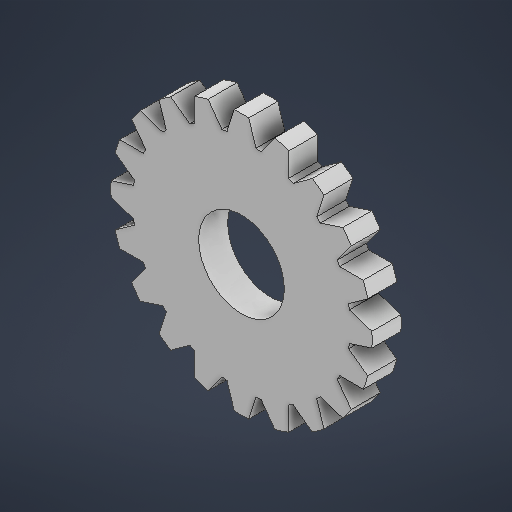
# Autodesk Inventor part: Engrenagem
Saved by Autodesk Inventor 2026.2 (Build 302298010, 298A)
## iProperties
Created: 2026-04-22
Part Number: Engrenagem
Material: Generic
Document SubType Name: Modeling
Designer: mrcm
Density: 1 g/cm^3
Appearance: Default
Author: mrcm
Autodesk Inventor part; units mm, degrees
ref_plane "YZ Plane" through (0, 0, 0) normal (1, 0, 0) x (0, 1, 0)
ref_plane "XZ Plane" through (0, 0, 0) normal (0, 1, 0) x (-1, 0, 0)
ref_plane "XY Plane" through (0, 0, 0) normal (0, 0, 1) x (1, 0, 0)
sketch "Sketch1" plane through (0, 0, 0) normal (0, 0, 1) x (1, 0, 0)
  arc A0 (12.7, 228.2469) -> (-12.7, 228.2469) centre (0, 0) ccw
  line L0 (-25.4, 188.7991) -> (-12.7, 228.2469)
  line L1 (12.7, 228.2469) -> (25.4, 188.7991)
  arc A1 (-58.4538, 221.0003) -> (-82.6106, 213.1512) centre (0, 0) ccw
  line L2 (-82.499, 171.7096) -> (-82.6106, 213.1512)
  line L3 (-58.4538, 221.0003) -> (-34.1853, 187.4076)
  arc A2 (-123.8857, 192.1205) -> (-144.4347, 177.1908) centre (0, 0) ccw
  line L4 (-131.5223, 137.8119) -> (-144.4347, 177.1908)
  line L5 (-123.8857, 192.1205) -> (-90.4243, 167.6714)
  arc A3 (-177.1908, 144.4347) -> (-192.1205, 123.8857) centre (0, 0) ccw
  line L6 (-167.6714, 90.4243) -> (-192.1205, 123.8857)
  line L7 (-177.1908, 144.4347) -> (-137.8119, 131.5223)
  arc A4 (-213.1512, 82.6106) -> (-221.0003, 58.4538) centre (0, 0) ccw
  line L8 (-187.4076, 34.1853) -> (-221.0003, 58.4538)
  line L9 (-213.1512, 82.6106) -> (-171.7096, 82.499)
  arc A5 (-228.2469, 12.7) -> (-228.2469, -12.7) centre (0, 0) ccw
  line L10 (-188.7991, -25.4) -> (-228.2469, -12.7)
  line L11 (-228.2469, 12.7) -> (-188.7991, 25.4)
  arc A6 (-221.0003, -58.4538) -> (-213.1512, -82.6106) centre (0, 0) ccw
  line L12 (-171.7096, -82.499) -> (-213.1512, -82.6106)
  line L13 (-221.0003, -58.4538) -> (-187.4076, -34.1853)
  arc A7 (-192.1205, -123.8857) -> (-177.1908, -144.4347) centre (0, 0) ccw
  line L14 (-137.8119, -131.5223) -> (-177.1908, -144.4347)
  line L15 (-192.1205, -123.8857) -> (-167.6714, -90.4243)
  arc A8 (-144.4347, -177.1908) -> (-123.8857, -192.1205) centre (0, 0) ccw
  line L16 (-90.4243, -167.6714) -> (-123.8857, -192.1205)
  line L17 (-144.4347, -177.1908) -> (-131.5223, -137.8119)
  arc A9 (-82.6106, -213.1512) -> (-58.4538, -221.0003) centre (0, 0) ccw
  line L18 (-34.1853, -187.4076) -> (-58.4538, -221.0003)
  line L19 (-82.6106, -213.1512) -> (-82.499, -171.7096)
  arc A10 (-12.7, -228.2469) -> (12.7, -228.2469) centre (0, 0) ccw
  line L20 (25.4, -188.7991) -> (12.7, -228.2469)
  line L21 (-12.7, -228.2469) -> (-25.4, -188.7991)
  arc A11 (58.4538, -221.0003) -> (82.6106, -213.1512) centre (0, 0) ccw
  line L22 (82.499, -171.7096) -> (82.6106, -213.1512)
  line L23 (58.4538, -221.0003) -> (34.1853, -187.4076)
  arc A12 (123.8857, -192.1205) -> (144.4347, -177.1908) centre (0, 0) ccw
  line L24 (131.5223, -137.8119) -> (144.4347, -177.1908)
  line L25 (123.8857, -192.1205) -> (90.4243, -167.6714)
  arc A13 (177.1908, -144.4347) -> (192.1205, -123.8857) centre (0, 0) ccw
  line L26 (167.6714, -90.4243) -> (192.1205, -123.8857)
  line L27 (177.1908, -144.4347) -> (137.8119, -131.5223)
  arc A14 (213.1512, -82.6106) -> (221.0003, -58.4538) centre (0, 0) ccw
  line L28 (187.4076, -34.1853) -> (221.0003, -58.4538)
  line L29 (213.1512, -82.6106) -> (171.7096, -82.499)
  arc A15 (228.2469, -12.7) -> (228.2469, 12.7) centre (0, 0) ccw
  line L30 (188.7991, 25.4) -> (228.2469, 12.7)
  line L31 (228.2469, -12.7) -> (188.7991, -25.4)
  arc A16 (221.0003, 58.4538) -> (213.1512, 82.6106) centre (0, 0) ccw
  line L32 (171.7096, 82.499) -> (213.1512, 82.6106)
  line L33 (221.0003, 58.4538) -> (187.4076, 34.1853)
  arc A17 (192.1205, 123.8857) -> (177.1908, 144.4347) centre (0, 0) ccw
  line L34 (137.8119, 131.5223) -> (177.1908, 144.4347)
  line L35 (192.1205, 123.8857) -> (167.6714, 90.4243)
  arc A18 (144.4347, 177.1908) -> (123.8857, 192.1205) centre (0, 0) ccw
  line L36 (90.4243, 167.6714) -> (123.8857, 192.1205)
  line L37 (144.4347, 177.1908) -> (131.5223, 137.8119)
  arc A19 (82.6106, 213.1512) -> (58.4538, 221.0003) centre (0, 0) ccw
  line L38 (34.1853, 187.4076) -> (58.4538, 221.0003)
  line L39 (82.6106, 213.1512) -> (82.499, 171.7096)
  arc A20 (-131.5223, 137.8119) -> (-137.8119, 131.5223) centre (0, 0) ccw
  arc A21 (-167.6714, 90.4243) -> (-171.7096, 82.499) centre (0, 0) ccw
  arc A22 (-187.4076, 34.1853) -> (-188.7991, 25.4) centre (0, 0) ccw
  arc A23 (-188.7991, -25.4) -> (-187.4076, -34.1853) centre (0, 0) ccw
  arc A24 (-171.7096, -82.499) -> (-167.6714, -90.4243) centre (0, 0) ccw
  arc A25 (-82.499, 171.7096) -> (-90.4243, 167.6714) centre (0, 0) ccw
  arc A26 (-25.4, 188.7991) -> (-34.1853, 187.4076) centre (0, 0) ccw
  arc A27 (34.1853, 187.4076) -> (25.4, 188.7991) centre (0, 0) ccw
  arc A28 (90.4243, 167.6714) -> (82.499, 171.7096) centre (0, 0) ccw
  arc A29 (137.8119, 131.5223) -> (131.5223, 137.8119) centre (0, 0) ccw
  arc A30 (171.7096, 82.499) -> (167.6714, 90.4243) centre (0, 0) ccw
  arc A31 (188.7991, 25.4) -> (187.4076, 34.1853) centre (0, 0) ccw
  arc A32 (187.4076, -34.1853) -> (188.7991, -25.4) centre (0, 0) ccw
  arc A33 (167.6714, -90.4243) -> (171.7096, -82.499) centre (0, 0) ccw
  arc A34 (131.5223, -137.8119) -> (137.8119, -131.5223) centre (0, 0) ccw
  arc A35 (82.499, -171.7096) -> (90.4243, -167.6714) centre (0, 0) ccw
  arc A36 (-137.8119, -131.5223) -> (-131.5223, -137.8119) centre (0, 0) ccw
  arc A37 (-90.4243, -167.6714) -> (-82.499, -171.7096) centre (0, 0) ccw
  arc A38 (-34.1853, -187.4076) -> (-25.4, -188.7991) centre (0, 0) ccw
  arc A39 (25.4, -188.7991) -> (34.1853, -187.4076) centre (0, 0) ccw
  circle A40 centre (0, 0) radius 75
  dimension "d10" = 457.2
  dimension "d18" = 360
  dimension "d20" = 150
  constraints: 80 end point, 80 point on circle, 41 centre point, 2 coincident, 161 other
  measures "d10" diameter of A0
  measures "d20" diameter of A40
extrude "Extrusion1" add sketch "Sketch1" along normal blind 50.8
body "Solid1"
